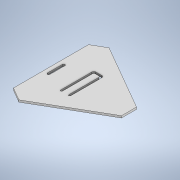
# Autodesk Inventor part: PCB_Bottom
Saved by Autodesk Inventor 2020.2 (Build 242310000, 310)
## iProperties
Created: 2021-02-25
Part Number: PCB_Bottom
Material: Generic
Document SubType Name: Modeling
Designer: saika
Density: 1 g/cm^3
Appearance: Default
Author: saika
Autodesk Inventor part; units mm, degrees
ref_plane "YZ Plane" through (0, 0, 0) normal (1, 0, 0) x (0, 1, 0)
ref_plane "XZ Plane" through (0, 0, 0) normal (0, 1, 0) x (-1, 0, 0)
ref_plane "XY Plane" through (0, 0, 0) normal (0, 0, 1) x (1, 0, 0)
sketch "Sketch1" plane through (0, 0, 0) normal (0, 1, 0) x (-1, 0, 0)
  line L0 (-38.1051, 6) -> (13.8564, 36)
  line L1 (-38.1051, -6) -> (13.8564, -36)
  line L2 (24.2487, 30) -> (24.2487, -30)
  line L3 (24.2487, 30) -> (13.8564, 36)
  line L4 (24.2487, -30) -> (13.8564, -36)
  line L5 (-38.1051, 6) -> (-38.1051, -6)
  line L6 (19.0526, 6) -> (19.0526, -6)
  line L7 (21.0526, -6) -> (21.0526, 6)
  arc A0 (21.0526, 6) -> (19.0526, 6) centre (20.0526, 6) ccw
  arc A1 (19.0526, -6) -> (21.0526, -6) centre (20.0526, -6) ccw
  line L8 (-2.5, 12.5) -> (-2.5, -11.5)
  line L9 (-1.5, -12.5) -> (1.5, -12.5)
  line L10 (2.5, -11.5) -> (2.5, 12.5)
  line L11 (-4, 12.5) -> (-4, -12.5)
  line L12 (-2.5, -14) -> (2.5, -14)
  line L13 (4, -12.5) -> (4, 12.5)
  arc A2 (4, 12.5) -> (2.5, 12.5) centre (3.25, 12.5) ccw
  arc A3 (-2.5, 12.5) -> (-4, 12.5) centre (-3.25, 12.5) ccw
  arc A4 (2.5, -14) -> (4, -12.5) centre (2.5, -12.5) ccw
  arc A5 (-4, -12.5) -> (-2.5, -14) centre (-2.5, -12.5) ccw
  arc A6 (-2.5, -11.5) -> (-1.5, -12.5) centre (-1.5, -11.5) ccw
  arc A7 (1.5, -12.5) -> (2.5, -11.5) centre (1.5, -11.5) ccw
  point P0 (0, 0)
  point P1 (0, 0)
  constraints: 28 end point, 16 point on circle, 15 tangent, 8 centre point, 2 equal radius, 2 parallel, 1 vertical
extrude "Extrusion1" add sketch "Sketch1" along normal blind 1.6
body "Solid1"
